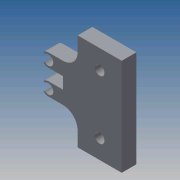
# Autodesk Inventor part: headphonesclip
Saved by Autodesk Inventor 2015 (Build 190159000, 159)
## iProperties
Created: 2015-09-02
Part Number: headphonesclip
Material: Generic
Document SubType Name: Modeling
Designer: Solomon
Density: 1 g/cm^3
Appearance: Default
Author: Solomon
Autodesk Inventor part; units mm, degrees
note: some values were not read from the file. Chosen so that the rebuilt part matches the saved one: sketch regions of "Extrusion3".
ref_plane "YZ Plane" through (0, 0, 0) normal (1, 0, 0) x (0, 1, 0)
ref_plane "XZ Plane" through (0, 0, 0) normal (0, 1, 0) x (-1, 0, 0)
ref_plane "XY Plane" through (0, 0, 0) normal (0, 0, 1) x (1, 0, 0)
sketch "Sketch1" plane through (0, 0, 0) normal (0, 1, 0) x (-1, 0, 0)
  arc A0 (1.2021, 1.2021) -> (1.2021, -1.2021) centre (0, 0) ccw
  arc A1 (1.591, 1.591) -> (1.591, -1.591) centre (0, 0) ccw
  line L0 (0, 2.25) -> (0, 1.7)
  line L1 (0, -1.7) -> (0, -2.25)
  line L2 (0, 0) -> (1.2021, -1.2021)
  line L3 (0, 0) -> (1.7, 0) construction
  line L4 (0, 0) -> (1.2021, 1.2021)
  line L5 (1.2021, -1.2021) -> (1.591, -1.591)
  line L6 (1.2021, 1.2021) -> (1.591, 1.591)
  line L7 (0, 2.25) -> (-5, 2.25)
  line L8 (-5, 2.25) -> (-5, -2.25)
  line L9 (-5, -2.25) -> (0, -2.25)
  line L10 (0, 0) -> (0, -8.5)
  arc A2 (1.2021, -7.2979) -> (1.2021, -9.7021) centre (0, -8.5) ccw
  arc A3 (1.591, -6.909) -> (1.591, -10.091) centre (0, -8.5) ccw
  line L11 (0, -8.5) -> (1.2021, -9.7021)
  line L12 (0, -8.5) -> (1.7, -8.5) construction
  line L13 (0, -8.5) -> (1.2021, -7.2979)
  line L14 (0, -8.5) -> (1.7, -8.5) construction
  line L15 (1.2021, -9.7021) -> (1.591, -10.091)
  line L16 (1.2021, -7.2979) -> (1.591, -6.909)
  line L17 (0, -6.25) -> (-5, -6.25)
  line L18 (0, -10.75) -> (-5, -10.75)
  line L19 (-5, -10.75) -> (-5, -6.25)
  line L20 (-5, -2.25) -> (-5, -6.25)
  line L21 (0, -2.25) -> (-5, -2.25)
  line L22 (-5, -2.25) -> (-5, -6.25)
  line L23 (-5, -6.25) -> (0, -6.25)
  line L24 (0, -6.25) -> (0, -2.25)
  arc A4 (-10, 7.25) -> (-5, 2.25) centre (-5, 7.25) ccw
  arc A5 (-5, -10.75) -> (-10, -15.75) centre (-5, -15.75) ccw
  line L25 (-10, -15.75) -> (-10, -20.75)
  line L26 (-10, 7.25) -> (-10, 12.25)
  line L27 (-10, -20.75) -> (-25, -20.75)
  line L28 (-10, 12.25) -> (-25, 12.25)
  line L29 (-25, 12.25) -> (-25, -20.75)
  line L30 (-5, -4.25) -> (-17.5, -4.25)
  line L31 (-17.5, -4.25) -> (-17.5, -14.25)
  line L32 (-17.5, -4.25) -> (-17.5, 5.75)
  circle A6 centre (-17.5, 5.75) radius 1.65
  circle A7 centre (-17.5, -14.25) radius 1.65
  dimension "d0" = 3.4
  dimension "d1" = 4.5
  dimension "d2" = 45
  dimension "d5" = 5
  dimension "d6" = 8.5
  dimension "d7" = 3.4
  dimension "d8" = 4.5
  dimension "d9" = 45
  dimension "d10" = 45
  dimension "d15" = 5
  dimension "d16" = 5
  dimension "d17" = 15
  dimension "d18" = 15
  dimension "d19" = 10
  dimension "d20" = 10
  dimension "d21" = 3.3
  dimension "d22" = 3.3
  constraints: 66 end point, 18 point on circle, 9 horizontal, 8 centre point, 7 vertical, 6 coincident, 6 perpendicular, 3 equal length, 3 tangent, 2 parallel, 1 collinear, 1 midpoint, 1 point on line
  measures "d0" diameter of A0
  measures "d1" diameter of A1
  measures "d2" angle of L2 L3
  measures "d5" distance of L0.start L7.end
  measures "d6" distance of L2.start L10.end
  measures "d7" diameter of A2
  measures "d8" diameter of A3
  measures "d9" angle of L11 L12
  measures "d10" angle of L14 L13
  measures "d15" distance of L25.start L25.end
  measures "d16" distance of L26.start L26.end
  measures "d17" distance of L25.end L27.end
  measures "d18" distance of L26.end L28.end
  measures "d19" distance of L30.end L31.end
  measures "d20" distance of L30.end L32.end
  measures "d21" diameter of A6
  measures "d22" diameter of A7
extrude "Extrusion3" add sketch "Sketch1" along normal blind 5 contours A0 L0 A1 L6 | A0 L1 A1 L0 | A0 L5 A1 L1 | A1 L9 L8 L7 | L8 L20 L19 A5 L25 L27 L29 L28 L26 A4 | A3 L16 A2 L10 | L10 A2 L15 A3 | A3 L18 L19 L17
body "Solid3"
